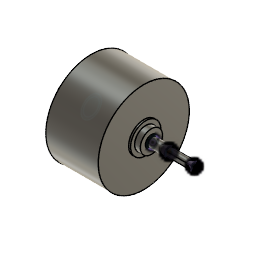
Motor (Autodesk Fusion 360 design; units mm, degrees)
part number: 2026-01-29-11-21-38-177
part number: 2026-01-29-12-04-20-137
part number: 2026-01-29-21-41-47-689
part number: 2026-01-29-21-45-58-319
Autodesk Fusion 360 part; units mm, degrees
ref_plane "WorkPlane1" through (0, 0, 0) normal (1, 0, 0) x (0, 1, 0) in component "Motor_Axis"
sketch "Sketch1" plane through (0, 0, 0) normal (1, 0, 0) x (0, 1, 0) in component "Motor_Axis"
  circle A0 centre (0, 0) radius 7.5
  circle A1 centre (0, 0) radius 9.5
  dimension "d3" = 15
  dimension "d17" = 19
  constraint coincident A0.centre A1.centre
  measures "d3" diameter of A0
  measures "d17" diameter of A1
extrude "Extrude1" add sketch "Sketch1" along normal blind 26 contours A0 makes body 1 in component "Motor_Axis"
sketch "Sketch3" plane through (26, 0, 0) normal (1, 0, 0) x (0, 1, 0) in component "Motor_Axis"
  circle A0 centre (0, 0) radius 7.5
  line L0 (-5, 3.3166) -> (-5, -3.3166)
  line L1 (5, -3.3166) -> (5, 3.3166)
  line L2 (5, 3.3166) -> (-5, -3.3166) construction
  line L3 (-5, 3.3166) -> (5, -3.3166) construction
  arc A1 (-5, -3.3166) -> (5, -3.3166) centre (0, 0) ccw
  arc A2 (5, 3.3166) -> (-5, 3.3166) centre (0, 0) ccw
  dimension "d9" = 12
  dimension "d10" = 10
  constraint coincident A0.centre A1.centre
  constraint parallel L0 L1
  constraint coincident L2 A0.centre
  constraint coincident L3 A0.centre
  constraint coincident L1.end A1
  constraint concentric A1 A2
  measures "d9" diameter of A1
  measures "d10" distance of L0.end L1.start
extrude "Extrude3" add sketch "Sketch3" along normal blind 40 contours L0 L1 A1 A2 bodies 1 in component "Motor_Axis"
sketch "Sketch4" plane through (66, 0, 0) normal (1, 0, 0) x (0, 1, 0) in component "Motor_Axis"
  arc A0 (5, 3.3166) -> (-5, 3.3166) centre (0, 0) ccw
  line L0 (-5, 3.3166) -> (-5, -3.3166)
  arc A1 (-5, -3.3166) -> (5, -3.3166) centre (0, 0) ccw
  line L1 (5, -3.3166) -> (5, 3.3166)
  circle A2 centre (0, 0) radius 3.75
  dimension "d13" = 7.5
  constraint coincident A0.centre A1.centre
  measures "d13" diameter of A2
extrude "Extrude4" cut sketch "Sketch4" against normal blind 66 contours A2 bodies 1 in component "Motor_Axis"
extrude "Extrude5" add sketch "Sketch1" against normal blind 2 separate body makes body 2 in component "Motor_Axis"
sketch "Sketch7" plane through (-2, 0, 0) normal (-1, 0, 0) x (0, -1, 0) in component "Motor_Axis"
  circle A0 centre (0, 0) radius 7.5
  circle A1 centre (0, 0) radius 9.5
  circle A2 centre (0, 0) radius 17.5
  dimension "d20" = 35
  constraint coincident A0.centre A1.centre
  measures "d20" diameter of A2
extrude "Extrude6" add sketch "Sketch7" along normal blind 9 separate body contours A2 makes body 3 in component "Motor_Axis"
sketch "Sketch8" plane through (-11, 0, 0) normal (-1, 0, 0) x (0, -1, 0) in component "Motor_Axis"
  circle A0 centre (0, 0) radius 9.5
  circle A1 centre (0, 0) radius 17.5
  circle A2 centre (0, 0) radius 24
  dimension "d23" = 48
  constraint coincident A0.centre A1.centre
  measures "d23" diameter of A2
extrude "Extrude7" add sketch "Sketch8" along normal blind 3 separate body contours A2 makes body 4 in component "Motor_Axis"
ref_plane "WorkPlane3" through (0, 0, 0) normal (0, 1, 0) x (0, 0, 1) in component "Motor_Axis"
sketch "Sketch9" plane through (0, 0, 0) normal (0, 1, 0) x (1, 0, 0) in component "Motor_Axis"
  line L0 (-14, -17.5) -> (-14, 17.5) construction
  line L1 (-152.0697, 0) -> (347.9303, 0) construction
  line L2 (-14, 0) -> (-14, -72)
  line L3 (-14, -72) -> (-97, -72)
  line L4 (-97, -72) -> (-97, 0)
  line L5 (-97, 0) -> (-14, 0)
  point P0 (-144, 0)
  point P1 (66, 0)
  point P2 (-14, 0)
  dimension "d27" = 500
  dimension "d28" = 210
  dimension "d42" = 83
  dimension "d43" = 72
  constraint perpendicular L0 L1
  constraint coincident L1 origin
  constraint coincident L1 P0
  constraint coincident P2 L2.start
  constraint perpendicular L1 L2
  constraint perpendicular L2 L3
  constraint coincident L1 L4.end
  constraint perpendicular L1 L4
  measures "d27" distance of L1.start L1.end
  measures "d28" distance of P0 P1
  measures "d42" distance of L2.end L3.end
  measures "d43" distance of L3.end L4.end
ref_plane "WorkPlane4" through (-144, 0, 0) normal (1, 0, 0) x (0, 1, 0) in component "Motor_Axis"
sketch "Sketch12" plane through (-144, 0, 0) normal (1, 0, 0) x (0, 1, 0) in component "Motor_Axis"
  circle A0 centre (0, 0) radius 6
  dimension "d30" = 12
  constraint coincident A0.centre origin
  measures "d30" diameter of A0
extrude "Extrude8" add sketch "Sketch12" along normal blind 33 separate body makes body 5 in component "Motor_Axis"
sketch "Sketch13" plane through (-111, 0, 0) normal (1, 0, 0) x (0, 1, 0) in component "Motor_Axis"
  circle A0 centre (0, 0) radius 6
  circle A1 centre (0, 0) radius 7.5
  dimension "d33" = 15
  constraint concentric A0 A1
  measures "d33" diameter of A1
extrude "Extrude9" add sketch "Sketch13" along normal blind 10 separate body makes body 6 in component "Motor_Axis"
sketch "Sketch14" plane through (-111, 0, 0) normal (1, 0, 0) x (0, 1, 0) in component "Motor_Axis"
  circle A0 centre (0, 0) radius 6
  circle A1 centre (0, 0) radius 12.5
  circle A2 centre (0, 0) radius 16.5
  dimension "d36" = 25
  dimension "d38" = 33
  constraint coincident A0.centre A1.centre
  constraint concentric A1 A2
  measures "d36" diameter of A1
  measures "d38" diameter of A2
extrude "Extrude10" add sketch "Sketch14" along normal blind 7 from surface at 7 separate body contours A2 makes body 7 in component "Motor_Axis"
sketch "Sketch16" plane through (-97, 0, 0) normal (1, 0, 0) x (0, 1, 0) in component "Motor_Axis"
  circle A0 centre (0, 0) radius 12.5
  circle A1 centre (0, 0) radius 16.5
revolve "Revolve1" add sketch "Sketch9" angle 360 about axis through (-152.0697, 0, 0) along (1, 0, 0) bodies 4 7 in component "Motor_Axis"
copy_body "CutPasteBodies1" bodies 2 removing the originals makes body 8 in component "ComponentMotor"
copy_body "CutPasteBodies2" bodies 3 removing the originals makes body 9 in component "ComponentMotor"
copy_body "CutPasteBodies3" bodies 4 removing the originals makes body 10 in component "ComponentMotor"
copy_body "CutPasteBodies1'" bodies 1 removing the originals makes body 11 in component "ComponentAxis"
copy_body "CutPasteBodies2'" bodies 5 removing the originals makes body 12 in component "ComponentAxis"
copy_body "CutPasteBodies3'" bodies 6 removing the originals makes body 13 in component "ComponentAxis"
component "Motor_Axis" placed x (1, 0, 0) y (0, 1, 0) z (0, 0, 1) at (0, 0, 0)
component "ComponentMotor" placed x (1, 0, 0) y (0, 1, 0) z (0, 0, 1) at (0, 0, 0)
component "ComponentAxis" placed x (1, 0, 0) y (0, 1, 0) z (0, 0, 1) at (0, 0, 0)
equation "BaseOffset = 0 mm" comment "work ofset axis from ORIGIN"
equation "d2 = BaseOffset"
equation "d26 = BaseOffset"
equation "d43 = 65 mm + 7 mm"
